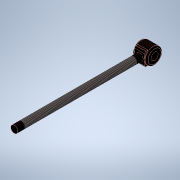
# Autodesk Inventor part: rod
Saved by Autodesk Inventor 2021 (Build 250183000, 183)
## iProperties
Created: 2021-07-29
Part Number: rod
Material: Generic
Document SubType Name: Modeling
Designer: Shammy Haider
Density: 1 g/cm^3
Appearance: Default
Author: Shammy Haider
Autodesk Inventor part; units mm, degrees
ref_plane "YZ Plane" through (0, 0, 0) normal (1, 0, 0) x (0, 1, 0)
ref_plane "XZ Plane" through (0, 0, 0) normal (0, 1, 0) x (-1, 0, 0)
sketch "Sketch1" plane through (0, 0, 0) normal (0, 0, 1) x (1, 0, 0)
  circle A0 centre (0, 0) radius 5
  dimension "d0" = 10
  constraints: 1 centre point, 1 coincident
  measures "d0" diameter of A0
extrude "Extrusion1" add sketch "Sketch1" along normal blind 180
thread "Thread1" size "M10x1.5" class "6g" standard "ANSI Metric M Profile" length 160 offset 10
sketch "Sketch2" plane through (0, 0, 0) normal (1, 0, 0) x (0, 1, 0)
  circle A0 centre (0, -9.9047) radius 11.3732
  point P0 (0, 0)
  constraints: 1 centre point
extrude "Extrusion2" add sketch "Sketch2" along normal mid plane 20
sketch "Sketch3" plane through (10, 0, -9.9047) normal (1, 0, 0) x (0, 0, -1)
  circle A0 centre (0, 0) radius 5
  point P0 (-9.9047, 0)
  dimension "d7" = 10
  constraints: 1 centre point
  measures "d7" diameter of A0
extrude "Extrusion3" cut sketch "Sketch3" against normal blind 20
fillet "Fillet1" radius 2 2 edges at (10, -11.3732, -9.9047) (-10, -11.3732, -9.9047)
ref_plane "Work Plane1" through (0, 0, 1.4685) normal (0, 0, 1) x (1, 0, 0)
sketch "Sketch4" plane through (0, 0, 1.4685) normal (0, 0, 1) x (1, 0, 0)
  line L0 (-7.1456, 9.3732) -> (7.1456, 9.3732)
  line L1 (7.1456, 9.3732) -> (7.1456, -9.3732)
  line L2 (7.1456, -9.3732) -> (-7.1456, -9.3732)
  line L3 (-7.1456, -9.3732) -> (-7.1456, 9.3732)
  line L4 (-7.1456, 9.3732) -> (7.1456, -9.3732) construction
  line L5 (7.1456, 9.3732) -> (-7.1456, -9.3732) construction
  point P0 (0, 0)
  constraints: 12 end point, 2 midpoint, 2 parallel, 1 horizontal, 1 perpendicular
extrude "Extrusion4" add sketch "Sketch4" against normal blind 5
fillet "Fillet2" radius 2 2 edges at (0, 9.3732, 1.4685) (0, -9.3732, 1.4685)
body "Solid1"
